Autodesk Fusion 360 part; units mm, degrees
note: some values were not read from the file. Chosen so that the rebuilt part matches the saved one: which bodies a step acts on; a direction. Set by a fixed rule: which sketch regions a step uses.
(part 4 of 5)
move_body "Move3'" bodies 154 to x (-1, 0, 0) y (0, -0.34202, 0.939693) z (0, 0.939693, 0.34202) at (3.0712, -87.9464, 93) in component "Camera cage R"
combine "Combine1''" operation add target body 152 tool bodies 153 154 in component "Camera cage R"
sketch "Cage flange R sketch" plane through (0, 0, 0) normal (0, 0, 1) x (1, 0, 0) in component "Camera cage R"
  line L0 (-30, -5.5) -> (30, -5.5)
  line L1 (30, -5.5) -> (30, 5.5)
  line L2 (30, 5.5) -> (-30, 5.5)
  line L3 (-30, 5.5) -> (-30, -5.5)
extrude "Cage flange R" add sketch "Cage flange R sketch" along normal blind 3 from surface at 8 separate body makes body 155 in component "Camera cage R"
move_body "Move4'" bodies 155 to x (-1, 0, 0) y (0, -0.34202, 0.939693) z (0, 0.939693, 0.34202) at (3.0712, -87.9464, 93) in component "Camera cage R"
combine "Combine2''" operation add target body 152 tool bodies 155 in component "Camera cage R"
sketch "Cage barrel opening R sketch" plane through (0, 0, 0) normal (0, 0, 1) x (1, 0, 0) in component "Camera cage R"
  circle A0 centre (0, 0) radius 8.5
extrude "Cage barrel opening R" add sketch "Cage barrel opening R sketch" along normal blind 5 from surface at 7 separate body makes body 156 in component "Camera cage R"
move_body "Move5'" bodies 156 to x (-1, 0, 0) y (0, -0.34202, 0.939693) z (0, 0.939693, 0.34202) at (3.0712, -87.9464, 93) in component "Camera cage R"
combine "Combine3'" operation cut target body 152 tool bodies 156 in component "Camera cage R"
sketch "Cage pilots R sketch" plane through (0, 0, 0) normal (0, 0, 1) x (1, 0, 0) in component "Camera cage R"
  line L0 (0.9, -15.8) -> (2.9, -15.8)
  line L1 (2.9, -15.8) -> (2.9, -13.8)
  line L2 (2.9, -13.8) -> (0.9, -13.8)
  line L3 (0.9, -13.8) -> (0.9, -15.8)
  line L4 (0.9, 13.7) -> (2.9, 13.7)
  line L5 (2.9, 13.7) -> (2.9, 15.7)
  line L6 (2.9, 15.7) -> (0.9, 15.7)
  line L7 (0.9, 15.7) -> (0.9, 13.7)
  line L8 (-4.2, -16.4) -> (-2.2, -16.4)
  line L9 (-2.2, -16.4) -> (-2.2, -14.4)
  line L10 (-2.2, -14.4) -> (-4.2, -14.4)
  line L11 (-4.2, -14.4) -> (-4.2, -16.4)
  line L12 (-4.2, 14.5) -> (-2.2, 14.5)
  line L13 (-2.2, 14.5) -> (-2.2, 16.5)
  line L14 (-2.2, 16.5) -> (-4.2, 16.5)
  line L15 (-4.2, 16.5) -> (-4.2, 14.5)
extrude "Cage pilots R" add sketch "Cage pilots R sketch" along normal blind 4.8 from surface at 22.8 separate body makes body 157 at (-4.2, -15.0667, 26) makes body 158 at (0.9, 15.0333, 26) makes body 159 at (0.9, -14.4667, 26) makes body 160 at (-4.2, 15.8333, 26) in component "Camera cage R"
move_body "Move6'" bodies 157 to x (-1, 0, 0) y (0, -0.34202, 0.939693) z (0, 0.939693, 0.34202) at (3.0712, -87.9464, 93) in component "Camera cage R"
move_body "Move7'" bodies 158 to x (-1, 0, 0) y (0, -0.34202, 0.939693) z (0, 0.939693, 0.34202) at (3.0712, -87.9464, 93) in component "Camera cage R"
move_body "Move8'" bodies 159 to x (-1, 0, 0) y (0, -0.34202, 0.939693) z (0, 0.939693, 0.34202) at (3.0712, -87.9464, 93) in component "Camera cage R"
move_body "Move9'" bodies 160 to x (-1, 0, 0) y (0, -0.34202, 0.939693) z (0, 0.939693, 0.34202) at (3.0712, -87.9464, 93) in component "Camera cage R"
combine "Combine4'" operation cut target body 152 tool bodies 157 158 159 160 in component "Camera cage R"
sketch "Cage ears R sketch" plane through (0, 0, 0) normal (0, 0, 1) x (1, 0, 0) in component "Camera cage R"
  line L0 (23.0712, -83.7036) -> (33.0712, -83.7036)
  line L1 (33.0712, -83.7036) -> (33.0712, -80)
  line L2 (33.0712, -80) -> (23.0712, -80)
  line L3 (23.0712, -80) -> (23.0712, -83.7036)
  line L4 (-26.9288, -85.8769) -> (-16.9288, -85.8769)
  line L5 (-16.9288, -85.8769) -> (-16.9288, -80)
  line L6 (-16.9288, -80) -> (-26.9288, -80)
  line L7 (-26.9288, -80) -> (-26.9288, -85.8769)
extrude "Cage ears R" add sketch "Cage ears R sketch" along normal blind 10 from surface at 90 separate body makes body 161 at (29.7378, -80, 93.3333) makes body 162 at (-20.2622, -80, 93.3333) in component "Camera cage R"
combine "Combine5'" operation add target body 152 tool bodies 161 162 in component "Camera cage R"
sketch "Cage M3 hole +1 sketch (2)" plane through (0, 0, 0) normal (0, 0, 1) x (1, 0, 0) in component "Camera cage R"
  line L0 (26.4712, -83.7036) -> (29.6712, -83.7036)
  line L1 (29.6712, -83.7036) -> (29.6712, -74.7036)
  line L2 (29.6712, -74.7036) -> (26.4712, -74.7036)
  line L3 (26.4712, -74.7036) -> (26.4712, -83.7036)
extrude "Cage M3 hole +1'" cut sketch "Cage M3 hole +1 sketch (2)" along normal blind 3.2 from surface at 93.4 bodies 152 in component "Camera cage R"
sketch "Cage M3 hole -1 sketch (2)" plane through (0, 0, 0) normal (0, 0, 1) x (1, 0, 0) in component "Camera cage R"
  line L0 (-23.5288, -85.8769) -> (-20.3288, -85.8769)
  line L1 (-20.3288, -85.8769) -> (-20.3288, -76.8769)
  line L2 (-20.3288, -76.8769) -> (-23.5288, -76.8769)
  line L3 (-23.5288, -76.8769) -> (-23.5288, -85.8769)
extrude "Cage M3 hole -1'" cut sketch "Cage M3 hole -1 sketch (2)" along normal blind 3.2 from surface at 93.4 bodies 152 in component "Camera cage R"
sketch "Lid plate sketch" plane through (0, 0, 0) normal (0, 0, 1) x (1, 0, 0) in component "Lid"
  circle A0 centre (0, 0) radius 105
extrude "Lid plate" add sketch "Lid plate sketch" along normal blind 3 from surface at 117 separate body makes body 163 in component "Lid"
sketch "Camera hump sketch" plane through (0, 0, 0) normal (0, 0, 1) x (1, 0, 0) in component "Lid"
  line L0 (-15, 54) -> (49, 54)
  line L1 (49, 54) -> (49, 79)
  line L2 (49, 79) -> (-15, 79)
  line L3 (-15, 79) -> (-15, 54)
extrude "Camera hump" add sketch "Camera hump sketch" along normal blind 5.5 from surface at 119.5 bodies 163 in component "Lid"
sketch "Camera hump sketch (1)" plane through (0, 0, 0) normal (0, 0, 1) x (1, 0, 0) in component "Lid"
  line L0 (-15, -79) -> (49, -79)
  line L1 (49, -79) -> (49, -54)
  line L2 (49, -54) -> (-15, -54)
  line L3 (-15, -54) -> (-15, -79)
extrude "Camera hump (1)" add sketch "Camera hump sketch (1)" along normal blind 5.5 from surface at 119.5 bodies 163 in component "Lid"
sketch "Camera pocket sketch" plane through (0, 0, 0) normal (0, 0, 1) x (1, 0, 0) in component "Lid"
  line L0 (-13, 56) -> (47, 56)
  line L1 (47, 56) -> (47, 77)
  line L2 (47, 77) -> (-13, 77)
  line L3 (-13, 77) -> (-13, 56)
extrude "Camera pocket" cut sketch "Camera pocket sketch" along normal blind 7 from surface at 116 bodies 163 in component "Lid"
sketch "Camera pocket sketch (1)" plane through (0, 0, 0) normal (0, 0, 1) x (1, 0, 0) in component "Lid"
  line L0 (-13, -77) -> (47, -77)
  line L1 (47, -77) -> (47, -56)
  line L2 (47, -56) -> (-13, -56)
  line L3 (-13, -56) -> (-13, -77)
extrude "Camera pocket (1)" cut sketch "Camera pocket sketch (1)" along normal blind 7 from surface at 116 bodies 163 in component "Lid"
sketch "Handle slot sketch" plane through (0, 0, 0) normal (0, 0, 1) x (1, 0, 0) in component "Lid"
  line L0 (29.5, -9) -> (90.5, -9)
  line L1 (90.5, -9) -> (90.5, 9)
  line L2 (90.5, 9) -> (29.5, 9)
  line L3 (29.5, 9) -> (29.5, -9)
extrude "Handle slot" cut sketch "Handle slot sketch" along normal blind 5 from surface at 116 bodies 163 in component "Lid"
sketch "Front notch sketch" plane through (0, 0, 0) normal (0, 0, 1) x (1, 0, 0) in component "Lid"
  line L0 (49, 7) -> (92, 7)
  line L1 (92, 7) -> (92, 35)
  line L2 (92, 35) -> (49, 35)
  line L3 (49, 35) -> (49, 7)
extrude "Front notch" cut sketch "Front notch sketch" along normal blind 5 from surface at 116 bodies 163 in component "Lid"
sketch "Finger notch sketch" plane through (0, 0, 0) normal (0, 0, 1) x (1, 0, 0) in component "Lid"
  line L0 (97.4603, 17.6488) -> (105.2855, 19.3121)
  line L1 (105.2855, 19.3121) -> (104.0381, 25.181)
  line L2 (104.0381, 25.181) -> (96.2129, 23.5177)
  line L3 (96.2129, 23.5177) -> (97.4603, 17.6488)
extrude "Finger notch" cut sketch "Finger notch sketch" along normal blind 5 from surface at 116 bodies 163 in component "Lid"
sketch "Finger notch sketch (1)" plane through (0, 0, 0) normal (0, 0, 1) x (1, 0, 0) in component "Lid"
  line L0 (96.2129, -23.5177) -> (104.0381, -25.181)
  line L1 (104.0381, -25.181) -> (105.2855, -19.3121)
  line L2 (105.2855, -19.3121) -> (97.4603, -17.6488)
  line L3 (97.4603, -17.6488) -> (96.2129, -23.5177)
extrude "Finger notch (1)" cut sketch "Finger notch sketch (1)" along normal blind 5 from surface at 116 bodies 163 in component "Lid"
sketch "Hook skirt +71 sketch" plane through (0, 0, 0) normal (0, 0, 1) x (1, 0, 0) in component "Lid"
  arc A0 (43.5428, 95.5459) -> (24.5118, 102.0988) centre (0, 0) ccw
  line L0 (24.5118, 102.0988) -> (24.1383, 100.543)
  arc A1 (42.8793, 94.09) -> (24.1383, 100.543) centre (0, 0) ccw
  line L1 (42.8793, 94.09) -> (43.5428, 95.5459)
extrude "Hook skirt +71" add sketch "Hook skirt +71 sketch" along normal blind 8.5 from surface at 109 bodies 163 in component "Lid"
sketch "Hook bump +71 sketch" plane through (0, 0, 0) normal (0, 0, 1) x (1, 0, 0) in component "Lid"
  arc A0 (41.3104, 95.0074) -> (25.9394, 100.3001) centre (0, 0) ccw
  line L0 (25.9394, 100.3001) -> (25.6389, 99.1383)
  arc A1 (40.8319, 93.907) -> (25.6389, 99.1383) centre (0, 0) ccw
  line L1 (40.8319, 93.907) -> (41.3104, 95.0074)
extrude "Hook bump +71" add sketch "Hook bump +71 sketch" along normal blind 3 from surface at 110.5 separate body makes body 164 in component "Lid"
sketch "Hook skirt +114 sketch" plane through (0, 0, 0) normal (0, 0, 1) x (1, 0, 0) in component "Lid"
  arc A0 (-33.317, 99.574) -> (-51.7045, 91.3873) centre (0, 0) ccw
  line L0 (-51.7045, 91.3873) -> (-50.9166, 89.9948)
  arc A1 (-32.8093, 98.0567) -> (-50.9166, 89.9948) centre (0, 0) ccw
  line L1 (-32.8093, 98.0567) -> (-33.317, 99.574)
extrude "Hook skirt +114" add sketch "Hook skirt +114 sketch" along normal blind 8.5 from surface at 109 bodies 163 in component "Lid"
sketch "Hook bump +114 sketch" plane through (0, 0, 0) normal (0, 0, 1) x (1, 0, 0) in component "Lid"
  arc A0 (-34.5824, 97.6577) -> (-49.4336, 91.0455) centre (0, 0) ccw
  line L0 (-49.4336, 91.0455) -> (-48.8611, 89.9909)
  arc A1 (-34.1818, 96.5265) -> (-48.8611, 89.9909) centre (0, 0) ccw
  line L1 (-34.1818, 96.5265) -> (-34.5824, 97.6577)
extrude "Hook bump +114" add sketch "Hook bump +114 sketch" along normal blind 3 from surface at 110.5 separate body makes body 165 in component "Lid"
sketch "Hook skirt -71 sketch" plane through (0, 0, 0) normal (0, 0, 1) x (1, 0, 0) in component "Lid"
  arc A0 (24.5118, -102.0988) -> (43.5428, -95.5459) centre (0, 0) ccw
  line L0 (43.5428, -95.5459) -> (42.8793, -94.09)
  arc A1 (24.1383, -100.543) -> (42.8793, -94.09) centre (0, 0) ccw
  line L1 (24.1383, -100.543) -> (24.5118, -102.0988)
extrude "Hook skirt -71" add sketch "Hook skirt -71 sketch" along normal blind 8.5 from surface at 109 bodies 163 in component "Lid"
sketch "Hook bump -71 sketch" plane through (0, 0, 0) normal (0, 0, 1) x (1, 0, 0) in component "Lid"
  arc A0 (25.9394, -100.3001) -> (41.3104, -95.0074) centre (0, 0) ccw
  line L0 (41.3104, -95.0074) -> (40.8319, -93.907)
  arc A1 (25.6389, -99.1383) -> (40.8319, -93.907) centre (0, 0) ccw
  line L1 (25.6389, -99.1383) -> (25.9394, -100.3001)
extrude "Hook bump -71" add sketch "Hook bump -71 sketch" along normal blind 3 from surface at 110.5 separate body makes body 166 in component "Lid"
sketch "Hook skirt -114 sketch" plane through (0, 0, 0) normal (0, 0, 1) x (1, 0, 0) in component "Lid"
  arc A0 (-51.7045, -91.3873) -> (-33.317, -99.574) centre (0, 0) ccw
  line L0 (-33.317, -99.574) -> (-32.8093, -98.0567)
  arc A1 (-50.9166, -89.9948) -> (-32.8093, -98.0567) centre (0, 0) ccw
  line L1 (-50.9166, -89.9948) -> (-51.7045, -91.3873)
extrude "Hook skirt -114" add sketch "Hook skirt -114 sketch" along normal blind 8.5 from surface at 109 bodies 163 in component "Lid"
sketch "Hook bump -114 sketch" plane through (0, 0, 0) normal (0, 0, 1) x (1, 0, 0) in component "Lid"
  arc A0 (-49.4336, -91.0455) -> (-34.5824, -97.6577) centre (0, 0) ccw
  line L0 (-34.5824, -97.6577) -> (-34.1818, -96.5265)
  arc A1 (-48.8611, -89.9909) -> (-34.1818, -96.5265) centre (0, 0) ccw
  line L1 (-48.8611, -89.9909) -> (-49.4336, -91.0455)
extrude "Hook bump -114" add sketch "Hook bump -114 sketch" along normal blind 3 from surface at 110.5 separate body makes body 167 in component "Lid"
sketch "Handle bar sketch" plane through (0, 0, 0) normal (0, 0, 1) x (1, 0, 0) in component "Handle bar"
  line L0 (33, -8) -> (87, -8)
  line L1 (87, -8) -> (87, 8)
  line L2 (87, 8) -> (33, 8)
  line L3 (33, 8) -> (33, -8)
extrude "Handle bar" add sketch "Handle bar sketch" along normal blind 16 from surface at 140 separate body makes body 168 in component "Handle bar"
sketch "Victim LED sketch" plane through (0, 0, 0) normal (0, 0, 1) x (1, 0, 0) in component "Victim LED"
  circle A0 centre (83.5, 0) radius 2.5
extrude "Victim LED" add sketch "Victim LED sketch" along normal blind 4 from surface at 156 separate body makes body 169 in component "Victim LED"
sketch "Start button sketch" plane through (0, 0, 0) normal (0, 0, 1) x (1, 0, 0) in component "Start button"
  circle A0 centre (75.5, 21.5) radius 6
extrude "Start button" add sketch "Start button sketch" along normal blind 7 from surface at 90 separate body makes body 170 in component "Start button"
sketch "Power switch sketch" plane through (0, 0, 0) normal (0, 0, 1) x (1, 0, 0) in component "Power switch"
  line L0 (53.5, 12) -> (66.5, 12)
  line L1 (66.5, 12) -> (66.5, 31)
  line L2 (66.5, 31) -> (53.5, 31)
  line L3 (53.5, 31) -> (53.5, 12)
extrude "Power switch" add sketch "Power switch sketch" along normal blind 13 from surface at 90 separate body makes body 171 in component "Power switch"
sketch "Status LED 1 sketch" plane through (0, 0, 0) normal (0, 0, 1) x (1, 0, 0) in component "Status LED 1"
  circle A0 centre (75, 0) radius 2
extrude "Status LED 1" add sketch "Status LED 1 sketch" along normal blind 4 from surface at 98 separate body makes body 172 in component "Status LED 1"
sketch "Status LED 2 sketch" plane through (0, 0, 0) normal (0, 0, 1) x (1, 0, 0) in component "Status LED 2"
  circle A0 centre (66, 0) radius 2
extrude "Status LED 2" add sketch "Status LED 2 sketch" along normal blind 4 from surface at 98 separate body makes body 173 in component "Status LED 2"
sketch "USB-C service socket sketch" plane through (0, 0, 0) normal (0, 0, 1) x (1, 0, 0) in component "USB-C service socket"
  line L0 (80.9456, -43.1544) -> (92.8217, -48.442)
  line L1 (92.8217, -48.442) -> (98.1093, -36.5659)
  line L2 (98.1093, -36.5659) -> (86.2332, -31.2784)
  line L3 (86.2332, -31.2784) -> (80.9456, -43.1544)
extrude "USB-C service socket" add sketch "USB-C service socket sketch" along normal blind 7 from surface at 71.5 separate body makes body 174 in component "USB-C service socket"
sketch "Dropper floor sketch" plane through (0, 0, 0) normal (0, 0, 1) x (1, 0, 0) in component "Dropper floor"
  circle A0 centre (-20, 0) radius 51.1342
extrude "Dropper floor" add sketch "Dropper floor sketch" along normal blind 3 from surface at 87 separate body makes body 175 in component "Dropper floor"
sketch "Dropper floor tab 0 sketch" plane through (0, 0, 0) normal (0, 0, 1) x (1, 0, 0) in component "Dropper floor"
  line L0 (30, 8.5) -> (39, 8.5)
  line L1 (39, 8.5) -> (39, 12.5)
  line L2 (39, 12.5) -> (30, 12.5)
  line L3 (30, 12.5) -> (30, 8.5)
extrude "Dropper floor tab 0" add sketch "Dropper floor tab 0 sketch" along normal blind 1.5 from surface at 88.5 bodies 175 in component "Dropper floor"
sketch "Dropper floor tab 1 sketch" plane through (0, 0, 0) normal (0, 0, 1) x (1, 0, 0) in component "Dropper floor"
  line L0 (30, -12.5) -> (39, -12.5)
  line L1 (39, -12.5) -> (39, -8.5)
  line L2 (39, -8.5) -> (30, -8.5)
  line L3 (30, -8.5) -> (30, -12.5)
extrude "Dropper floor tab 1" add sketch "Dropper floor tab 1 sketch" along normal blind 1.5 from surface at 88.5 bodies 175 in component "Dropper floor"
sketch "Dropper floor tab 2 sketch" plane through (0, 0, 0) normal (0, 0, 1) x (1, 0, 0) in component "Dropper floor"
  line L0 (-75, -5) -> (-69, -5)
  line L1 (-69, -5) -> (-69, 5)
  line L2 (-69, 5) -> (-75, 5)
  line L3 (-75, 5) -> (-75, -5)
extrude "Dropper floor tab 2" add sketch "Dropper floor tab 2 sketch" along normal blind 1.5 from surface at 88.5 bodies 175 in component "Dropper floor"
sketch "Slot A sketch" plane through (0, 0, 0) normal (0, 0, 1) x (1, 0, 0) in component "Dropper floor"
  line L0 (-47.2943, -39.3151) -> (-35.2735, -27.2943)
  line L1 (-35.2735, -27.2943) -> (-47.2943, -15.2735)
  line L2 (-47.2943, -15.2735) -> (-59.3151, -27.2943)
  line L3 (-59.3151, -27.2943) -> (-47.2943, -39.3151)
extrude "Slot A" cut sketch "Slot A sketch" along normal blind 5 from surface at 86 bodies 175 in component "Dropper floor"
sketch "Slot B sketch" plane through (0, 0, 0) normal (0, 0, 1) x (1, 0, 0) in component "Dropper floor"
  line L0 (-47.2943, 15.2735) -> (-35.2735, 27.2943)
  line L1 (-35.2735, 27.2943) -> (-47.2943, 39.3151)
  line L2 (-47.2943, 39.3151) -> (-59.3151, 27.2943)
  line L3 (-59.3151, 27.2943) -> (-47.2943, 15.2735)
extrude "Slot B" cut sketch "Slot B sketch" along normal blind 5 from surface at 86 bodies 175 in component "Dropper floor"
sketch "N20 pocket sketch" plane through (0, 0, 0) normal (0, 0, 1) x (1, 0, 0) in component "Dropper floor"
  line L0 (-25.2, -6.2) -> (-14.8, -6.2)
  line L1 (-14.8, -6.2) -> (-14.8, 6.2)
  line L2 (-14.8, 6.2) -> (-25.2, 6.2)
  line L3 (-25.2, 6.2) -> (-25.2, -6.2)
extrude "N20 pocket" cut sketch "N20 pocket sketch" along normal blind 5 from surface at 86 bodies 175 in component "Dropper floor"
sketch "N20 face plate recess sketch" plane through (0, 0, 0) normal (0, 0, 1) x (1, 0, 0) in component "Dropper floor"
  line L0 (-28.2, -9.2) -> (-11.8, -9.2)
  line L1 (-11.8, -9.2) -> (-11.8, 9.2)
  line L2 (-11.8, 9.2) -> (-28.2, 9.2)
  line L3 (-28.2, 9.2) -> (-28.2, -9.2)
extrude "N20 face plate recess" cut sketch "N20 face plate recess sketch" along normal blind 3 from surface at 88 bodies 175 in component "Dropper floor"
sketch "Dropper plate sketch" plane through (0, 0, 0) normal (0, 0, 1) x (1, 0, 0) in component "Dropper plate"
  circle A0 centre (-20, 0) radius 49.1342
extrude "Dropper plate" add sketch "Dropper plate sketch" along normal blind 12 from surface at 90 separate body makes body 176 in component "Dropper plate"
sketch "Pocket 1 sketch" plane through (0, 0, 0) normal (0, 0, 1) x (1, 0, 0) in component "Dropper plate"
  line L0 (-34.5866, -29.3239) -> (-37.9513, -41.8809)
  line L1 (-37.9513, -41.8809) -> (-25.3942, -45.2456)
  line L2 (-25.3942, -45.2456) -> (-22.0296, -32.6885)
  line L3 (-22.0296, -32.6885) -> (-34.5866, -29.3239)
extrude "Pocket 1" cut sketch "Pocket 1 sketch" along normal blind 14 from surface at 89 bodies 176 in component "Dropper plate"
sketch "Pocket 2 sketch" plane through (0, 0, 0) normal (0, 0, 1) x (1, 0, 0) in component "Dropper plate"
  line L0 (-17.9704, -32.6885) -> (-14.6058, -45.2456)
  line L1 (-14.6058, -45.2456) -> (-2.0487, -41.8809)
  line L2 (-2.0487, -41.8809) -> (-5.4134, -29.3239)
  line L3 (-5.4134, -29.3239) -> (-17.9704, -32.6885)
extrude "Pocket 2" cut sketch "Pocket 2 sketch" along normal blind 14 from surface at 89 bodies 176 in component "Dropper plate"
sketch "Pocket 3 sketch" plane through (0, 0, 0) normal (0, 0, 1) x (1, 0, 0) in component "Dropper plate"
  line L0 (-1.8981, -27.2943) -> (7.2943, -36.4867)
  line L1 (7.2943, -36.4867) -> (16.4867, -27.2943)
  line L2 (16.4867, -27.2943) -> (7.2943, -18.1019)
  line L3 (7.2943, -18.1019) -> (-1.8981, -27.2943)
extrude "Pocket 3" cut sketch "Pocket 3 sketch" along normal blind 14 from surface at 89 bodies 176 in component "Dropper plate"
sketch "Pocket 4 sketch" plane through (0, 0, 0) normal (0, 0, 1) x (1, 0, 0) in component "Dropper plate"
  line L0 (9.3239, -14.5866) -> (21.8809, -17.9513)
  line L1 (21.8809, -17.9513) -> (25.2456, -5.3942)
  line L2 (25.2456, -5.3942) -> (12.6885, -2.0296)
  line L3 (12.6885, -2.0296) -> (9.3239, -14.5866)
extrude "Pocket 4" cut sketch "Pocket 4 sketch" along normal blind 14 from surface at 89 bodies 176 in component "Dropper plate"
sketch "Pocket 5 sketch" plane through (0, 0, 0) normal (0, 0, 1) x (1, 0, 0) in component "Dropper plate"
  line L0 (12.6885, 2.0296) -> (25.2456, 5.3942)
  line L1 (25.2456, 5.3942) -> (21.8809, 17.9513)
  line L2 (21.8809, 17.9513) -> (9.3239, 14.5866)
  line L3 (9.3239, 14.5866) -> (12.6885, 2.0296)
extrude "Pocket 5" cut sketch "Pocket 5 sketch" along normal blind 14 from surface at 89 bodies 176 in component "Dropper plate"
sketch "Pocket 6 sketch" plane through (0, 0, 0) normal (0, 0, 1) x (1, 0, 0) in component "Dropper plate"
  line L0 (7.2943, 18.1019) -> (16.4867, 27.2943)
  line L1 (16.4867, 27.2943) -> (7.2943, 36.4867)
  line L2 (7.2943, 36.4867) -> (-1.8981, 27.2943)
  line L3 (-1.8981, 27.2943) -> (7.2943, 18.1019)
extrude "Pocket 6" cut sketch "Pocket 6 sketch" along normal blind 14 from surface at 89 bodies 176 in component "Dropper plate"
sketch "Pocket 7 sketch" plane through (0, 0, 0) normal (0, 0, 1) x (1, 0, 0) in component "Dropper plate"
  line L0 (-5.4134, 29.3239) -> (-2.0487, 41.8809)
  line L1 (-2.0487, 41.8809) -> (-14.6058, 45.2456)
  line L2 (-14.6058, 45.2456) -> (-17.9704, 32.6885)
  line L3 (-17.9704, 32.6885) -> (-5.4134, 29.3239)
extrude "Pocket 7" cut sketch "Pocket 7 sketch" along normal blind 14 from surface at 89 bodies 176 in component "Dropper plate"
sketch "Pocket 8 sketch" plane through (0, 0, 0) normal (0, 0, 1) x (1, 0, 0) in component "Dropper plate"
  line L0 (-22.0296, 32.6885) -> (-25.3942, 45.2456)
  line L1 (-25.3942, 45.2456) -> (-37.9513, 41.8809)
  line L2 (-37.9513, 41.8809) -> (-34.5866, 29.3239)
  line L3 (-34.5866, 29.3239) -> (-22.0296, 32.6885)
extrude "Pocket 8" cut sketch "Pocket 8 sketch" along normal blind 14 from surface at 89 bodies 176 in component "Dropper plate"
sketch "Shaft bore sketch (5)" plane through (0, 0, 0) normal (0, 0, 1) x (1, 0, 0) in component "Dropper plate"
  circle A0 centre (-20, 0) radius 1.5
extrude "Shaft bore''''" cut sketch "Shaft bore sketch (5)" along normal blind 14 from surface at 89 bodies 176 in component "Dropper plate"
sketch "N20 gearmotor with encoder sketch" plane through (0, 0, 0) normal (0, 0, 1) x (1, 0, 0) in component "N20 motor"
  line L0 (-25, -6) -> (-15, -6)
  line L1 (-15, -6) -> (-15, 6)
  line L2 (-15, 6) -> (-25, 6)
  line L3 (-25, 6) -> (-25, -6)
extrude "N20 gearmotor with encoder" add sketch "N20 gearmotor with encoder sketch" along normal blind 41.5 from surface at 46.5 separate body makes body 177 in component "N20 motor"
sketch "N20 shaft sketch" plane through (0, 0, 0) normal (0, 0, 1) x (1, 0, 0) in component "N20 motor"
  circle A0 centre (-20, 0) radius 1.5
extrude "N20 shaft" add sketch "N20 shaft sketch" along normal blind 10 from surface at 88 separate body makes body 178 in component "N20 motor"
sketch "N20 face plate sketch" plane through (0, 0, 0) normal (0, 0, 1) x (1, 0, 0) in component "N20 face plate"
  line L0 (-28, -9) -> (-12, -9)
  line L1 (-12, -9) -> (-12, 9)
  line L2 (-12, 9) -> (-28, 9)
  line L3 (-28, 9) -> (-28, -9)
extrude "N20 face plate" add sketch "N20 face plate sketch" along normal blind 2 from surface at 88 separate body makes body 179 in component "N20 face plate"
sketch "Shaft bore sketch (6)" plane through (0, 0, 0) normal (0, 0, 1) x (1, 0, 0) in component "N20 face plate"
  circle A0 centre (-20, 0) radius 1.7
extrude "Shaft bore'''''" cut sketch "Shaft bore sketch (6)" along normal blind 4 from surface at 87 bodies 179 in component "N20 face plate"
sketch "Kit 1 sketch" plane through (0, 0, 0) normal (0, 0, 1) x (1, 0, 0) in component "Kits"
  line L0 (-33.632, -30.9773) -> (-36.2979, -40.9263)
  line L1 (-36.2979, -40.9263) -> (-26.3488, -43.5922)
  line L2 (-26.3488, -43.5922) -> (-23.683, -33.6431)
  line L3 (-23.683, -33.6431) -> (-33.632, -30.9773)
extrude "Kit 1" add sketch "Kit 1 sketch" along normal blind 10.3 from surface at 90 separate body makes body 180 in component "Kits"
sketch "Kit 2 sketch" plane through (0, 0, 0) normal (0, 0, 1) x (1, 0, 0) in component "Kits"
  line L0 (-16.317, -33.6431) -> (-13.6512, -43.5922)
  line L1 (-13.6512, -43.5922) -> (-3.7021, -40.9263)
  line L2 (-3.7021, -40.9263) -> (-6.368, -30.9773)
  line L3 (-6.368, -30.9773) -> (-16.317, -33.6431)
extrude "Kit 2" add sketch "Kit 2 sketch" along normal blind 10.3 from surface at 90 separate body makes body 181 in component "Kits"
sketch "Kit 3 sketch" plane through (0, 0, 0) normal (0, 0, 1) x (1, 0, 0) in component "Kits"
  line L0 (0.0111, -27.2943) -> (7.2943, -34.5775)
  line L1 (7.2943, -34.5775) -> (14.5775, -27.2943)
  line L2 (14.5775, -27.2943) -> (7.2943, -20.0111)
  line L3 (7.2943, -20.0111) -> (0.0111, -27.2943)
extrude "Kit 3" add sketch "Kit 3 sketch" along normal blind 10.3 from surface at 90 separate body makes body 182 in component "Kits"
sketch "Kit 4 sketch" plane through (0, 0, 0) normal (0, 0, 1) x (1, 0, 0) in component "Kits"
  line L0 (10.9773, -13.632) -> (20.9263, -16.2979)
  line L1 (20.9263, -16.2979) -> (23.5922, -6.3488)
  line L2 (23.5922, -6.3488) -> (13.6431, -3.683)
  line L3 (13.6431, -3.683) -> (10.9773, -13.632)
extrude "Kit 4" add sketch "Kit 4 sketch" along normal blind 10.3 from surface at 90 separate body makes body 183 in component "Kits"
sketch "Kit 5 sketch" plane through (0, 0, 0) normal (0, 0, 1) x (1, 0, 0) in component "Kits"
  line L0 (13.6431, 3.683) -> (23.5922, 6.3488)
  line L1 (23.5922, 6.3488) -> (20.9263, 16.2979)
  line L2 (20.9263, 16.2979) -> (10.9773, 13.632)
  line L3 (10.9773, 13.632) -> (13.6431, 3.683)
extrude "Kit 5" add sketch "Kit 5 sketch" along normal blind 10.3 from surface at 90 separate body makes body 184 in component "Kits"
sketch "Kit 6 sketch" plane through (0, 0, 0) normal (0, 0, 1) x (1, 0, 0) in component "Kits"
  line L0 (7.2943, 20.0111) -> (14.5775, 27.2943)
  line L1 (14.5775, 27.2943) -> (7.2943, 34.5775)
  line L2 (7.2943, 34.5775) -> (0.0111, 27.2943)
  line L3 (0.0111, 27.2943) -> (7.2943, 20.0111)
extrude "Kit 6" add sketch "Kit 6 sketch" along normal blind 10.3 from surface at 90 separate body makes body 185 in component "Kits"
sketch "Kit 7 sketch" plane through (0, 0, 0) normal (0, 0, 1) x (1, 0, 0) in component "Kits"
  line L0 (-6.368, 30.9773) -> (-3.7021, 40.9263)
  line L1 (-3.7021, 40.9263) -> (-13.6512, 43.5922)
  line L2 (-13.6512, 43.5922) -> (-16.317, 33.6431)
  line L3 (-16.317, 33.6431) -> (-6.368, 30.9773)
extrude "Kit 7" add sketch "Kit 7 sketch" along normal blind 10.3 from surface at 90 separate body makes body 186 in component "Kits"
sketch "Kit 8 sketch" plane through (0, 0, 0) normal (0, 0, 1) x (1, 0, 0) in component "Kits"
  line L0 (-23.683, 33.6431) -> (-26.3488, 43.5922)
  line L1 (-26.3488, 43.5922) -> (-36.2979, 40.9263)
  line L2 (-36.2979, 40.9263) -> (-33.632, 30.9773)
  line L3 (-33.632, 30.9773) -> (-23.683, 33.6431)
extrude "Kit 8" add sketch "Kit 8 sketch" along normal blind 10.3 from surface at 90 separate body makes body 187 in component "Kits"
sketch "Hopper sketch" plane through (0, 0, 0) normal (0, 0, 1) x (1, 0, 0) in component "Hopper B left"
  line L0 (-47.2943, 11.738) -> (-31.738, 27.2943)
  line L1 (-31.738, 27.2943) -> (-47.2943, 42.8507)
  line L2 (-47.2943, 42.8507) -> (-62.8507, 27.2943)
  line L3 (-62.8507, 27.2943) -> (-47.2943, 11.738)
extrude "Hopper" add sketch "Hopper sketch" along normal blind 15 from surface at 72 separate body makes body 188 in component "Hopper B left"
sketch "Hopper flange sketch" plane through (0, 0, 0) normal (0, 0, 1) x (1, 0, 0) in component "Hopper B left"
  line L0 (-47.2943, 8.9095) -> (-28.9095, 27.2943)
  line L1 (-28.9095, 27.2943) -> (-47.2943, 45.6791)
  line L2 (-47.2943, 45.6791) -> (-65.6791, 27.2943)
  line L3 (-65.6791, 27.2943) -> (-47.2943, 8.9095)
extrude "Hopper flange" add sketch "Hopper flange sketch" along normal blind 1.5 from surface at 85.5 bodies 188 in component "Hopper B left"
sketch "Hopper void sketch" plane through (0, 0, 0) normal (0, 0, 1) x (1, 0, 0) in component "Hopper B left"
  line L0 (-47.2943, 15.2735) -> (-35.2735, 27.2943)
  line L1 (-35.2735, 27.2943) -> (-47.2943, 39.3151)
  line L2 (-47.2943, 39.3151) -> (-59.3151, 27.2943)
  line L3 (-59.3151, 27.2943) -> (-47.2943, 15.2735)
extrude "Hopper void" cut sketch "Hopper void sketch" along normal blind 14.4 from surface at 73.6 bodies 188 in component "Hopper B left"
sketch "Socket tool sketch" plane through (0, 0, 0) normal (0, 0, 1) x (1, 0, 0) in component "Hopper B left"
  line L0 (-11.1, -9.6) -> (11.1, -9.6)
  line L1 (11.1, -9.6) -> (11.1, 20.6)
  line L2 (11.1, 20.6) -> (-11.1, 20.6)
  line L3 (-11.1, 20.6) -> (-11.1, -9.6)
extrude "Socket tool" add sketch "Socket tool sketch" along normal blind 35 separate body makes body 189 in component "Hopper B left"
move_body "Move1'''" bodies 189 to x (-0.977496, -0.210954, 0) y (-0.112564, 0.521586, 0.845741) z (-0.178413, 0.826708, -0.533594) at (-46.4023, 23.1608, 82.168) in component "Hopper B left"
combine "Combine1'''" operation cut target body 188 tool bodies 189 in component "Hopper B left"
sketch "Channel sketch" plane through (0, 0, 0) normal (0, 0, 1) x (1, 0, 0) in component "Chute B left"
  line L0 (-11.1, -9.6) -> (11.1, -9.6)
  line L1 (11.1, -9.6) -> (11.1, 12.6)
  line L2 (11.1, 12.6) -> (-11.1, 12.6)
  line L3 (-11.1, 12.6) -> (-11.1, -9.6)
extrude "Channel" add sketch "Channel sketch" along normal blind 79.2151 separate body makes body 190 in component "Chute B left"
move_body "Move1''''" bodies 190 to x (-0.977496, -0.210954, 0) y (-0.112564, 0.521586, 0.845741) z (-0.178413, 0.826708, -0.533594) at (-47.2943, 27.2943, 79.5) in component "Chute B left"
sketch "Channel void sketch" plane through (0, 0, 0) normal (0, 0, 1) x (1, 0, 0) in component "Chute B left"
  line L0 (-9.5, -8) -> (9.5, -8)
  line L1 (9.5, -8) -> (9.5, 11)
  line L2 (9.5, 11) -> (-9.5, 11)
  line L3 (-9.5, 11) -> (-9.5, -8)
extrude "Channel void" add sketch "Channel void sketch" along normal blind 83.2151 separate body makes body 191 in component "Chute B left"
move_body "Move2'''" bodies 191 to x (-0.977496, -0.210954, 0) y (-0.112564, 0.521586, 0.845741) z (-0.178413, 0.826708, -0.533594) at (-46.9375, 25.6409, 80.5672) in component "Chute B left"
combine "Combine1''''" operation cut target body 190 tool bodies 191 in component "Chute B left"
sketch "Trough cut sketch" plane through (0, 0, 0) normal (0, 0, 1) x (1, 0, 0) in component "Chute B left"
  line L0 (-47.2943, 9.6167) -> (-29.6167, 27.2943)
  line L1 (-29.6167, 27.2943) -> (-47.2943, 44.972)
  line L2 (-47.2943, 44.972) -> (-64.972, 27.2943)
  line L3 (-64.972, 27.2943) -> (-47.2943, 9.6167)
extrude "Trough cut" cut sketch "Trough cut sketch" along normal blind 40 from surface at 50 bodies 190 in component "Chute B left"
sketch "Floor slab sketch" plane through (0, 0, 0) normal (0, 0, 1) x (1, 0, 0) in component "Chute B left"
  line L0 (-11.1, -9.6) -> (11.1, -9.6)
  line L1 (11.1, -9.6) -> (11.1, -8)
  line L2 (11.1, -8) -> (-11.1, -8)
  line L3 (-11.1, -8) -> (-11.1, -9.6)
extrude "Floor slab" add sketch "Floor slab sketch" along normal blind 28 separate body makes body 192 in component "Chute B left"
move_body "Move3''" bodies 192 to x (-0.977496, -0.210954, 0) y (-0.112564, 0.521586, 0.845741) z (-0.178413, 0.826708, -0.533594) at (-47.2943, 27.2943, 79.5) in component "Chute B left"
combine "Combine2'''" operation add target body 190 tool bodies 192 in component "Chute B left"
sketch "Dropper floor clearance cut sketch" plane through (0, 0, 0) normal (0, 0, 1) x (1, 0, 0) in component "Chute B left"
  circle A0 centre (0, 0) radius 140
extrude "Dropper floor clearance cut" cut sketch "Dropper floor clearance cut sketch" along normal blind 10 from surface at 87 bodies 190 in component "Chute B left"
sketch "Trim sketch" plane through (0, 0, 0) normal (0, 0, 1) x (1, 0, 0) in component "Chute B left"
  circle A0 centre (0, 0) radius 140
  circle A1 centre (0, 0) radius 105
extrude "Trim" add sketch "Trim sketch" along normal blind 70 from surface at 20 separate body makes body 193 in component "Chute B left"
combine "Combine3''" operation cut target body 190 tool bodies 193 in component "Chute B left"
sketch "Hopper sketch (2)" plane through (0, 0, 0) normal (0, 0, 1) x (1, 0, 0) in component "Hopper A right"
  line L0 (-47.2943, -42.8507) -> (-31.738, -27.2943)
  line L1 (-31.738, -27.2943) -> (-47.2943, -11.738)
  line L2 (-47.2943, -11.738) -> (-62.8507, -27.2943)
  line L3 (-62.8507, -27.2943) -> (-47.2943, -42.8507)
extrude "Hopper'" add sketch "Hopper sketch (2)" along normal blind 15 from surface at 72 separate body makes body 194 in component "Hopper A right"
sketch "Hopper flange sketch (2)" plane through (0, 0, 0) normal (0, 0, 1) x (1, 0, 0) in component "Hopper A right"
  line L0 (-47.2943, -45.6791) -> (-28.9095, -27.2943)
  line L1 (-28.9095, -27.2943) -> (-47.2943, -8.9095)
  line L2 (-47.2943, -8.9095) -> (-65.6791, -27.2943)
  line L3 (-65.6791, -27.2943) -> (-47.2943, -45.6791)
extrude "Hopper flange'" add sketch "Hopper flange sketch (2)" along normal blind 1.5 from surface at 85.5 bodies 194 in component "Hopper A right"
sketch "Hopper void sketch (2)" plane through (0, 0, 0) normal (0, 0, 1) x (1, 0, 0) in component "Hopper A right"
  line L0 (-47.2943, -39.3151) -> (-35.2735, -27.2943)
  line L1 (-35.2735, -27.2943) -> (-47.2943, -15.2735)
  line L2 (-47.2943, -15.2735) -> (-59.3151, -27.2943)
  line L3 (-59.3151, -27.2943) -> (-47.2943, -39.3151)
extrude "Hopper void'" cut sketch "Hopper void sketch (2)" along normal blind 14.4 from surface at 73.6 bodies 194 in component "Hopper A right"
sketch "Socket tool sketch (2)" plane through (0, 0, 0) normal (0, 0, 1) x (1, 0, 0) in component "Hopper A right"
  line L0 (-11.1, -9.6) -> (11.1, -9.6)
  line L1 (11.1, -9.6) -> (11.1, 20.6)
  line L2 (11.1, 20.6) -> (-11.1, 20.6)
  line L3 (-11.1, 20.6) -> (-11.1, -9.6)
extrude "Socket tool'" add sketch "Socket tool sketch (2)" along normal blind 35 separate body makes body 195 in component "Hopper A right"
move_body "Move1'''''" bodies 195 to x (0.977496, -0.210954, 0) y (-0.112564, -0.521586, 0.845741) z (-0.178413, -0.826708, -0.533594) at (-46.4023, -23.1608, 82.168) in component "Hopper A right"
combine "Combine1'''''" operation cut target body 194 tool bodies 195 in component "Hopper A right"
sketch "Channel sketch (2)" plane through (0, 0, 0) normal (0, 0, 1) x (1, 0, 0) in component "Chute A right"
  line L0 (-11.1, -9.6) -> (11.1, -9.6)
  line L1 (11.1, -9.6) -> (11.1, 12.6)
  line L2 (11.1, 12.6) -> (-11.1, 12.6)
  line L3 (-11.1, 12.6) -> (-11.1, -9.6)
extrude "Channel'" add sketch "Channel sketch (2)" along normal blind 79.2151 separate body makes body 196 in component "Chute A right"
move_body "Move1''''''" bodies 196 to x (0.977496, -0.210954, 0) y (-0.112564, -0.521586, 0.845741) z (-0.178413, -0.826708, -0.533594) at (-47.2943, -27.2943, 79.5) in component "Chute A right"
sketch "Channel void sketch (2)" plane through (0, 0, 0) normal (0, 0, 1) x (1, 0, 0) in component "Chute A right"
  line L0 (-9.5, -8) -> (9.5, -8)
  line L1 (9.5, -8) -> (9.5, 11)
  line L2 (9.5, 11) -> (-9.5, 11)
  line L3 (-9.5, 11) -> (-9.5, -8)
extrude "Channel void'" add sketch "Channel void sketch (2)" along normal blind 83.2151 separate body makes body 197 in component "Chute A right"
move_body "Move2''''" bodies 197 to x (0.977496, -0.210954, 0) y (-0.112564, -0.521586, 0.845741) z (-0.178413, -0.826708, -0.533594) at (-46.9375, -25.6409, 80.5672) in component "Chute A right"
combine "Combine1''''''" operation cut target body 196 tool bodies 197 in component "Chute A right"
sketch "Trough cut sketch (2)" plane through (0, 0, 0) normal (0, 0, 1) x (1, 0, 0) in component "Chute A right"
  line L0 (-47.2943, -44.972) -> (-29.6167, -27.2943)
  line L1 (-29.6167, -27.2943) -> (-47.2943, -9.6167)
  line L2 (-47.2943, -9.6167) -> (-64.972, -27.2943)
  line L3 (-64.972, -27.2943) -> (-47.2943, -44.972)
extrude "Trough cut'" cut sketch "Trough cut sketch (2)" along normal blind 40 from surface at 50 bodies 196 in component "Chute A right"
sketch "Floor slab sketch (2)" plane through (0, 0, 0) normal (0, 0, 1) x (1, 0, 0) in component "Chute A right"
  line L0 (-11.1, -9.6) -> (11.1, -9.6)
  line L1 (11.1, -9.6) -> (11.1, -8)
  line L2 (11.1, -8) -> (-11.1, -8)
  line L3 (-11.1, -8) -> (-11.1, -9.6)
extrude "Floor slab'" add sketch "Floor slab sketch (2)" along normal blind 28 separate body makes body 198 in component "Chute A right"
move_body "Move3'''" bodies 198 to x (0.977496, -0.210954, 0) y (-0.112564, -0.521586, 0.845741) z (-0.178413, -0.826708, -0.533594) at (-47.2943, -27.2943, 79.5) in component "Chute A right"
combine "Combine2''''" operation add target body 196 tool bodies 198 in component "Chute A right"
sketch "Dropper floor clearance cut sketch (2)" plane through (0, 0, 0) normal (0, 0, 1) x (1, 0, 0) in component "Chute A right"
  circle A0 centre (0, 0) radius 140
extrude "Dropper floor clearance cut'" cut sketch "Dropper floor clearance cut sketch (2)" along normal blind 10 from surface at 87 bodies 196 in component "Chute A right"
sketch "Trim sketch (2)" plane through (0, 0, 0) normal (0, 0, 1) x (1, 0, 0) in component "Chute A right"
  circle A0 centre (0, 0) radius 140
  circle A1 centre (0, 0) radius 105
extrude "Trim'" add sketch "Trim sketch (2)" along normal blind 70 from surface at 20 separate body makes body 199 in component "Chute A right"
combine "Combine3'''" operation cut target body 196 tool bodies 199 in component "Chute A right"
sketch "GIGA post H1 sketch" plane through (0, 0, 0) normal (0, 0, 1) x (1, 0, 0) in component "GIGA posts"
  circle A0 centre (58.72, -16.17) radius 3.5
extrude "GIGA post H1" add sketch "GIGA post H1 sketch" along normal blind 22.5 from surface at 39 separate body makes body 200 in component "GIGA posts"
sketch "Insert hole H1 sketch" plane through (0, 0, 0) normal (0, 0, 1) x (1, 0, 0) in component "GIGA posts"
  circle A0 centre (58.72, -16.17) radius 2
extrude "Insert hole H1" cut sketch "Insert hole H1 sketch" along normal blind 7 from surface at 55.5 bodies 200 in component "GIGA posts"
sketch "GIGA post H2 sketch" plane through (0, 0, 0) normal (0, 0, 1) x (1, 0, 0) in component "GIGA posts"
  circle A0 centre (-16.21, -16.17) radius 3.5
extrude "GIGA post H2" add sketch "GIGA post H2 sketch" along normal blind 22.5 from surface at 39 separate body makes body 201 in component "GIGA posts"
sketch "Insert hole H2 sketch" plane through (0, 0, 0) normal (0, 0, 1) x (1, 0, 0) in component "GIGA posts"
  circle A0 centre (-16.21, -16.17) radius 2
extrude "Insert hole H2" cut sketch "Insert hole H2 sketch" along normal blind 7 from surface at 55.5 bodies 201 in component "GIGA posts"
sketch "GIGA post H3 sketch" plane through (0, 0, 0) normal (0, 0, 1) x (1, 0, 0) in component "GIGA posts"
  circle A0 centre (60.06, -64.33) radius 3.5
extrude "GIGA post H3" add sketch "GIGA post H3 sketch" along normal blind 22.5 from surface at 39 separate body makes body 202 in component "GIGA posts"
sketch "Insert hole H3 sketch" plane through (0, 0, 0) normal (0, 0, 1) x (1, 0, 0) in component "GIGA posts"
  circle A0 centre (60.06, -64.33) radius 2
extrude "Insert hole H3" cut sketch "Insert hole H3 sketch" along normal blind 7 from surface at 55.5 bodies 202 in component "GIGA posts"
sketch "GIGA post H4 sketch" plane through (0, 0, 0) normal (0, 0, 1) x (1, 0, 0) in component "GIGA posts"
  circle A0 centre (-22.74, -64.33) radius 3.5
extrude "GIGA post H4" add sketch "GIGA post H4 sketch" along normal blind 22.5 from surface at 39 separate body makes body 203 in component "GIGA posts"
sketch "Insert hole H4 sketch" plane through (0, 0, 0) normal (0, 0, 1) x (1, 0, 0) in component "GIGA posts"
  circle A0 centre (-22.74, -64.33) radius 2
extrude "Insert hole H4" cut sketch "Insert hole H4 sketch" along normal blind 7 from surface at 55.5 bodies 203 in component "GIGA posts"
sketch "GIGA board sketch" plane through (0, 0, 0) normal (0, 0, 1) x (1, 0, 0) in component "Arduino GIGA R1"
  line L0 (-27.56, -66.97) -> (73.96, -66.97)
  line L1 (73.96, -66.97) -> (73.96, -13.63)
  line L2 (73.96, -13.63) -> (-27.56, -13.63)
  line L3 (-27.56, -13.63) -> (-27.56, -66.97)
extrude "GIGA board" add sketch "GIGA board sketch" along normal blind 1.6 from surface at 61.5 separate body makes body 204 in component "Arduino GIGA R1"
sketch "Header strip +y sketch" plane through (0, 0, 0) normal (0, 0, 1) x (1, 0, 0) in component "Arduino GIGA R1"
  line L0 (-23.56, -17.38) -> (69.96, -17.38)
  line L1 (69.96, -17.38) -> (69.96, -14.88)
  line L2 (69.96, -14.88) -> (-23.56, -14.88)
  line L3 (-23.56, -14.88) -> (-23.56, -17.38)
extrude "Header strip +y" add sketch "Header strip +y sketch" along normal blind 8.5 from surface at 63.1 separate body makes body 205 in component "Arduino GIGA R1"
sketch "Header strip -y sketch" plane through (0, 0, 0) normal (0, 0, 1) x (1, 0, 0) in component "Arduino GIGA R1"
  line L0 (-23.56, -65.72) -> (69.96, -65.72)
  line L1 (69.96, -65.72) -> (69.96, -63.22)
  line L2 (69.96, -63.22) -> (-23.56, -63.22)
  line L3 (-23.56, -63.22) -> (-23.56, -65.72)
extrude "Header strip -y" add sketch "Header strip -y sketch" along normal blind 8.5 from surface at 63.1 separate body makes body 206 in component "Arduino GIGA R1"
sketch "Main PCB shield (placeholder) sketch" plane through (0, 0, 0) normal (0, 0, 1) x (1, 0, 0) in component "Main PCB"
  line L0 (-27.56, -66.97) -> (73.96, -66.97)
  line L1 (73.96, -66.97) -> (73.96, -13.63)
  line L2 (73.96, -13.63) -> (-27.56, -13.63)
  line L3 (-27.56, -13.63) -> (-27.56, -66.97)
extrude "Main PCB shield (placeholder)" add sketch "Main PCB shield (placeholder) sketch" along normal blind 1.6 from surface at 71.6 separate body makes body 207 in component "Main PCB"
sketch "PCB component envelope (placeholder) sketch" plane through (0, 0, 0) normal (0, 0, 1) x (1, 0, 0) in component "Main PCB"
  line L0 (-24.56, -63.97) -> (70.96, -63.97)
  line L1 (70.96, -63.97) -> (70.96, -16.63)
  line L2 (70.96, -16.63) -> (-24.56, -16.63)
  line L3 (-24.56, -16.63) -> (-24.56, -63.97)
extrude "PCB component envelope (placeholder)" add sketch "PCB component envelope (placeholder) sketch" along normal blind 7.3 from surface at 73.2 separate body makes body 208 in component "Main PCB"
sketch "Battery (placeholder 7.0 x 3.5 x 2.5) sketch" plane through (0, 0, 0) normal (0, 0, 1) x (1, 0, 0) in component "Battery"
  line L0 (7.5706, 20.1882) -> (76.5071, 32.3436)
  line L1 (76.5071, 32.3436) -> (70.4294, 66.8118)
  line L2 (70.4294, 66.8118) -> (1.4929, 54.6564)
  line L3 (1.4929, 54.6564) -> (7.5706, 20.1882)
extrude "Battery (placeholder 7.0 x 3.5 x 2.5)" add sketch "Battery (placeholder 7.0 x 3.5 x 2.5) sketch" along normal blind 25 from surface at 51 separate body makes body 209 in component "Battery"
sketch "Floor sensor FP (black, blue, red) sketch" plane through (0, 0, 0) normal (0, 0, 1) x (1, 0, 0) in component "Floor port FP"
  line L0 (64.85, 24.85) -> (85.15, 24.85)
  line L1 (85.15, 24.85) -> (85.15, 45.15)
  line L2 (85.15, 45.15) -> (64.85, 45.15)
  line L3 (64.85, 45.15) -> (64.85, 24.85)
extrude "Floor sensor FP (black, blue, red)" add sketch "Floor sensor FP (black, blue, red) sketch" along normal blind 14 from surface at 28 separate body makes body 210 in component "Floor port FP"
sketch "Silver module SM (straight + 20 deg tilted pair) sketch" plane through (0, 0, 0) normal (0, 0, 1) x (1, 0, 0) in component "Silver module SM"
  line L0 (65, -38) -> (85, -38)
  line L1 (85, -38) -> (85, -16)
  line L2 (85, -16) -> (65, -16)
  line L3 (65, -16) -> (65, -38)
extrude "Silver module SM (straight + 20 deg tilted pair)" add sketch "Silver module SM (straight + 20 deg tilted pair) sketch" along normal blind 14 from surface at 28 separate body makes body 211 in component "Silver module SM"
sketch "USB-C J12 sketch" plane through (0, 0, 0) normal (0, 0, 1) x (1, 0, 0) in component "Arduino GIGA R1"
  line L0 (72.96, -31.93) -> (76.96, -31.93)
  line L1 (76.96, -31.93) -> (76.96, -22.93)
  line L2 (76.96, -22.93) -> (72.96, -22.93)
  line L3 (72.96, -22.93) -> (72.96, -31.93)
extrude "USB-C J12" add sketch "USB-C J12 sketch" along normal blind 3.5 from surface at 63.1 separate body makes body 212 in component "Arduino GIGA R1"
sketch "Wi-Fi antenna sketch" plane through (0, 0, 0) normal (0, 0, 1) x (1, 0, 0) in component "Wi-Fi antenna"
  line L0 (92.3541, -40.7648) -> (92.8177, -40.9521)
  line L1 (92.8177, -40.9521) -> (95.2152, -35.0181)
  line L2 (95.2152, -35.0181) -> (94.7516, -34.8308)
  line L3 (94.7516, -34.8308) -> (92.3541, -40.7648)
extrude "Wi-Fi antenna" add sketch "Wi-Fi antenna sketch" along normal blind 15.4 from surface at 50 separate body makes body 213 in component "Wi-Fi antenna"
sketch "BNO055 board sketch" plane through (0, 0, 0) normal (0, 0, 1) x (1, 0, 0) in component "BNO055 IMU"
  line L0 (-63.5, -10) -> (-36.5, -10)
  line L1 (-36.5, -10) -> (-36.5, 10)
  line L2 (-36.5, 10) -> (-63.5, 10)
  line L3 (-63.5, 10) -> (-63.5, -10)
extrude "BNO055 board" add sketch "BNO055 board sketch" along normal blind 1.6 from surface at 44 separate body makes body 214 in component "BNO055 IMU"
sketch "Board holes sketch (12)" plane through (0, 0, 0) normal (0, 0, 1) x (1, 0, 0) in component "BNO055 IMU"
  line L0 (-41.25, 4.75) -> (-38.75, 4.75)
  line L1 (-38.75, 4.75) -> (-38.75, 7.25)
  line L2 (-38.75, 7.25) -> (-41.25, 7.25)
  line L3 (-41.25, 7.25) -> (-41.25, 4.75)
  line L4 (-41.25, -7.25) -> (-38.75, -7.25)
  line L5 (-38.75, -7.25) -> (-38.75, -4.75)
  line L6 (-38.75, -4.75) -> (-41.25, -4.75)
  line L7 (-41.25, -4.75) -> (-41.25, -7.25)
  line L8 (-61.25, 4.75) -> (-58.75, 4.75)
  line L9 (-58.75, 4.75) -> (-58.75, 7.25)
  line L10 (-58.75, 7.25) -> (-61.25, 7.25)
  line L11 (-61.25, 7.25) -> (-61.25, 4.75)
  line L12 (-61.25, -7.25) -> (-58.75, -7.25)
  line L13 (-58.75, -7.25) -> (-58.75, -4.75)
  line L14 (-58.75, -4.75) -> (-61.25, -4.75)
  line L15 (-61.25, -4.75) -> (-61.25, -7.25)
extrude "Board holes'''''''''''" cut sketch "Board holes sketch (12)" along normal blind 2.6 from surface at 43.5 bodies 214 in component "BNO055 IMU"
sketch "BNO055 chip sketch" plane through (0, 0, 0) normal (0, 0, 1) x (1, 0, 0) in component "BNO055 IMU"
  line L0 (-52.6, -1.9) -> (-47.4, -1.9)
  line L1 (-47.4, -1.9) -> (-47.4, 1.9)
  line L2 (-47.4, 1.9) -> (-52.6, 1.9)
  line L3 (-52.6, 1.9) -> (-52.6, -1.9)
extrude "BNO055 chip" add sketch "BNO055 chip sketch" along normal blind 1.1 from surface at 45.6 separate body makes body 215 in component "BNO055 IMU"
sketch "M2.5 screw heads sketch" plane through (0, 0, 0) normal (0, 0, 1) x (1, 0, 0) in component "BNO055 IMU"
  line L0 (-42.25, 3.75) -> (-37.75, 3.75)
  line L1 (-37.75, 3.75) -> (-37.75, 8.25)
  line L2 (-37.75, 8.25) -> (-42.25, 8.25)
  line L3 (-42.25, 8.25) -> (-42.25, 3.75)
  line L4 (-42.25, -8.25) -> (-37.75, -8.25)
  line L5 (-37.75, -8.25) -> (-37.75, -3.75)
  line L6 (-37.75, -3.75) -> (-42.25, -3.75)
  line L7 (-42.25, -3.75) -> (-42.25, -8.25)
  line L8 (-62.25, 3.75) -> (-57.75, 3.75)
  line L9 (-57.75, 3.75) -> (-57.75, 8.25)
  line L10 (-57.75, 8.25) -> (-62.25, 8.25)
  line L11 (-62.25, 8.25) -> (-62.25, 3.75)
  line L12 (-62.25, -8.25) -> (-57.75, -8.25)
  line L13 (-57.75, -8.25) -> (-57.75, -3.75)
  line L14 (-57.75, -3.75) -> (-62.25, -3.75)
  line L15 (-62.25, -3.75) -> (-62.25, -8.25)
extrude "M2.5 screw heads" add sketch "M2.5 screw heads sketch" along normal blind 1.5 from surface at 45.6 separate body makes body 216 at (-60.75, 5.25, 45.6) makes body 217 at (-40.75, -5.25, 45.6) makes body 218 at (-40.75, 6.75, 45.6) makes body 219 at (-60.75, -6.75, 45.6) in component "BNO055 IMU"
sketch "M2.5 screw shafts sketch" plane through (0, 0, 0) normal (0, 0, 1) x (1, 0, 0) in component "BNO055 IMU"
  line L0 (-40.95, 5.05) -> (-39.05, 5.05)
  line L1 (-39.05, 5.05) -> (-39.05, 6.95)
  line L2 (-39.05, 6.95) -> (-40.95, 6.95)
  line L3 (-40.95, 6.95) -> (-40.95, 5.05)
  line L4 (-40.95, -6.95) -> (-39.05, -6.95)
  line L5 (-39.05, -6.95) -> (-39.05, -5.05)
  line L6 (-39.05, -5.05) -> (-40.95, -5.05)
  line L7 (-40.95, -5.05) -> (-40.95, -6.95)
  line L8 (-60.95, 5.05) -> (-59.05, 5.05)
  line L9 (-59.05, 5.05) -> (-59.05, 6.95)
  line L10 (-59.05, 6.95) -> (-60.95, 6.95)
  line L11 (-60.95, 6.95) -> (-60.95, 5.05)
  line L12 (-60.95, -6.95) -> (-59.05, -6.95)
  line L13 (-59.05, -6.95) -> (-59.05, -5.05)
  line L14 (-59.05, -5.05) -> (-60.95, -5.05)
  line L15 (-60.95, -5.05) -> (-60.95, -6.95)
extrude "M2.5 screw shafts" add sketch "M2.5 screw shafts sketch" along normal blind 5.6 from surface at 40 separate body makes body 220 at (-60.95, 6.3167, 43.7333) makes body 221 at (-40.95, -5.6833, 43.7333) makes body 222 at (-40.95, 6.3167, 43.7333) makes body 223 at (-60.95, -5.6833, 43.7333) in component "BNO055 IMU"
sketch "Body sketch" plane through (0, 0, 0) normal (0, 0, 1) x (1, 0, 0) in component "Stepper bay 28BYJ-48"
  circle A0 centre (-14.8577, 6.1284) radius 14
extrude "Body" add sketch "Body sketch" along normal blind 19 from surface at 68 separate body makes body 224 in component "Stepper bay 28BYJ-48"